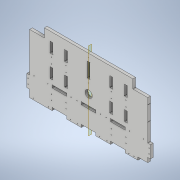
# Autodesk Inventor part: Side_one
Saved by Autodesk Inventor 2020 (Build 240168000, 168)
## iProperties
Created: 2019-12-17
Part Number: Side_one
Material: Generic
Document SubType Name: Modeling
Designer: fabfarm
Density: 1 g/cm^3
Appearance: Default
Author: fabfarm
Autodesk Inventor part; units mm, degrees
ref_plane "YZ Plane" through (0, 0, 0) normal (1, 0, 0) x (0, 1, 0)
ref_plane "XZ Plane" through (0, 0, 0) normal (0, 1, 0) x (-1, 0, 0)
ref_plane "XY Plane" through (0, 0, 0) normal (0, 0, 1) x (1, 0, 0)
sketch "Sketch1" plane through (0, 0, 0) normal (0, 0, 1) x (1, 0, 0)
  line L0 (0, 0) -> (-845, 0)
  line L1 (-845, 0) -> (-845, 464.3)
  line L2 (-845, 464.3) -> (0, 464.3)
  line L3 (0, 464.3) -> (0, 0)
  dimension "d0" = 464.3
  dimension "d1" = 845
  constraints: 8 end point, 2 parallel, 1 horizontal, 1 perpendicular
  measures "d0" distance of L2.end L0.start
  measures "d1" distance of L0.start L0.end
extrude "Extrusion1" add sketch "Sketch1" along normal blind 18.55
sketch "Sketch2" plane through (0, 0, 18.55) normal (0, 0, 1) x (1, 0, 0)
  line L0 (-845, 464.3) -> (-845, 0) projected
  line L1 (-845, 464.3) -> (-826.45, 464.3)
  line L2 (-826.45, 464.3) -> (-826.45, 359.9)
  line L3 (-826.45, 359.9) -> (-845, 359.9)
  line L4 (-845, 359.9) -> (-845, 464.3)
  line L5 (0, 464.3) -> (-845, 464.3) projected
  line L6 (-845, 259.9) -> (-826.45, 259.9)
  line L7 (-826.45, 259.9) -> (-826.45, 134.8)
  line L8 (-826.45, 134.8) -> (-845, 134.8)
  line L9 (-845, 134.8) -> (-845, 259.9)
  point P0 (-845, 359.9)
  point P1 (-845, 134.8)
  dimension "d54" = 18.55
  dimension "d55" = 104.4
  dimension "d86" = 100
  dimension "d87" = 125.1
  constraints: 16 end point, 4 parallel, 2 collinear, 2 horizontal, 2 perpendicular, 2 point on line
  measures "d54" distance of L1.start L1.end
  measures "d55" distance of L1.end L2.end
  measures "d86" distance between parallel lines of L6 L3
  measures "d87" distance of L6.end L7.end
extrude "Extrusion2" cut sketch "Sketch2" against normal blind 18.55
ref_plane "Work Plane1" through (-422.5, 259.9, 0) normal (-1, 0, 0) x (0, 0, 1)
mirror "Mirror1" about plane through (-422.5, 259.9, 0) normal (-1, 0, 0) of "Extrusion2"
sketch "Sketch3" plane through (0, 0, 18.55) normal (0, 0, 1) x (1, 0, 0)
  line L0 (0, 464.3) -> (-845, 464.3) projected
  line L1 (-845, 404.3) -> (-725, 404.3)
  line L2 (-725, 404.3) -> (-725, 464.3)
  line L3 (-725, 464.3) -> (-845, 464.3)
  line L4 (-845, 464.3) -> (-845, 404.3)
  point P0 (0, 0)
  point P1 (-18.55, 350)
  point P2 (0, 464.3)
  dimension "d19" = 120
  dimension "d22" = 60
  constraints: 8 end point, 2 perpendicular, 1 parallel, 2 other
  measures "d19" distance of L3.end L2.end
  measures "d22" distance of L3.end L1.start
extrude "Extrusion3" cut sketch "Sketch3" against normal blind 18.55
mirror "Mirror2" about plane through (-422.5, 259.9, 0) normal (-1, 0, 0) of "Extrusion3"
sketch "Sketch4" plane through (0, 0, 18.55) normal (0, 0, 1) x (1, 0, 0)
  line L0 (-672.5, 134.8) -> (-572.5, 134.8)
  line L1 (-572.5, 134.8) -> (-572.5, 153.35)
  line L2 (-572.5, 153.35) -> (-672.5, 153.35)
  line L3 (-672.5, 153.35) -> (-672.5, 134.8)
  line L4 (-472.5, 134.8) -> (-372.5, 134.8)
  line L5 (-372.5, 134.8) -> (-372.5, 153.35)
  line L6 (-372.5, 153.35) -> (-472.5, 153.35)
  line L7 (-472.5, 153.35) -> (-472.5, 134.8)
  line L8 (-272.5, 134.8) -> (-172.5, 134.8)
  line L9 (-172.5, 134.8) -> (-172.5, 153.35)
  line L10 (-172.5, 153.35) -> (-272.5, 153.35)
  line L11 (-272.5, 153.35) -> (-272.5, 134.8)
  line L12 (0, 0) -> (0, 359.9) projected
  line L13 (-845, 359.9) -> (-845, 0) projected
  line L14 (-826.45, 134.8) -> (-845, 134.8) projected
  line L15 (-845, 259.9) -> (-826.45, 259.9) projected
  line L16 (-120, 464.3) -> (-725, 464.3) projected
  line L17 (-422.5, 464.3) -> (-422.5, 153.35) construction
  dimension "d59" = 100
  dimension "d60" = 100
  dimension "d61" = 100
  dimension "d62" = 100
  dimension "d63" = 100
  dimension "d66" = 18.55
  constraints: 26 end point, 6 parallel, 5 collinear, 3 horizontal, 3 perpendicular, 2 midpoint, 1 vertical
  measures "d59" distance of L1.end L2.end
  measures "d60" distance of L5.end L6.end
  measures "d61" distance between parallel lines of L1 L7
  measures "d62" distance between parallel lines of L11 L5
  measures "d63" distance of L9.end L10.end
  measures "d66" distance of L2.end L0.start
extrude "Extrusion4" cut sketch "Sketch4" against normal blind 20
sketch "Sketch6" plane through (0, 0, 18.55) normal (0, 0, 1) x (1, 0, 0)
  line L0 (-372.5, 400.4) -> (-472.5, 400.4)
  line L1 (-472.5, 400.4) -> (-472.5, 425.4)
  line L2 (-472.5, 425.4) -> (-372.5, 425.4)
  line L3 (-372.5, 425.4) -> (-372.5, 400.4)
  line L4 (-372.5, 400.4) -> (-472.5, 425.4) construction
  line L5 (-472.5, 400.4) -> (-372.5, 425.4) construction
  line L6 (-422.5, -92.86) -> (-422.5, 557.16) projected
  line L7 (-120, 464.3) -> (-725, 464.3) projected
  point P0 (0, 0)
  point P1 (-422.5, 412.9)
  dimension "d38" = 25
  dimension "d39" = 100
  dimension "d40" = 38.9
  constraints: 12 end point, 2 midpoint, 2 parallel, 1 horizontal, 1 perpendicular, 1 point on line
  measures "d38" distance of L0.end L1.end
  measures "d39" distance of L1.end L2.end
  measures "d40" distance between parallel lines of L7 L2
extrude "Extrusion6" [suppressed]
fillet "Fillet1" [suppressed]
sketch "Sketch7" plane through (0, 0, 18.55) normal (0, 0, 1) x (1, 0, 0)
  line L0 (-686.45, 183.35) -> (-667.9, 183.35)
  line L1 (-667.9, 183.35) -> (-667.9, 253.85)
  line L2 (-667.9, 253.85) -> (-686.45, 253.85)
  line L3 (-686.45, 253.85) -> (-686.45, 183.35)
  line L4 (-586.5, 183.35) -> (-567.95, 183.35)
  line L5 (-567.95, 183.35) -> (-567.95, 253.85)
  line L6 (-567.95, 253.85) -> (-586.5, 253.85)
  line L7 (-586.5, 253.85) -> (-586.5, 183.35)
  line L8 (-725, 464.3) -> (-725, 404.3) projected
  line L9 (-672.5, 153.35) -> (-572.5, 153.35) projected
  line L10 (-826.45, 259.9) -> (-826.45, 134.8) projected
  point P0 (0, 0)
  dimension "d44" = 81.4
  dimension "d45" = 18.55
  dimension "d46" = 70.5
  dimension "d72" = 30
  dimension "d194" = 140
  constraints: 16 end point, 4 parallel, 2 horizontal, 2 perpendicular, 2 point on line, 1 collinear
  measures "d44" distance between parallel lines of L7 L1
  measures "d45" distance of L1.end L2.end
  measures "d46" distance of L2.end L0.start
  measures "d72" distance between parallel lines of L9 L0
  measures "d194" distance between parallel lines of L10 L3
extrude "Extrusion7" cut sketch "Sketch7" against normal blind 20
mirror "Mirror3" about plane through (-422.5, 259.9, 0) normal (-1, 0, 0) of "Extrusion7"
sketch "Esquisse8" plane through (0, 0, 0) normal (0, 0, -1) x (-1, 0, 0)
  line L0 (177.1, 334.35) -> (158.55, 334.35)
  line L1 (158.55, 334.35) -> (158.55, 404.85)
  line L2 (158.55, 404.85) -> (177.1, 404.85)
  line L3 (177.1, 404.85) -> (177.1, 334.35)
  line L4 (258.5, 404.85) -> (277.05, 404.85)
  line L5 (277.05, 404.85) -> (277.05, 334.35)
  line L6 (277.05, 334.35) -> (258.5, 334.35)
  line L7 (258.5, 334.35) -> (258.5, 404.85)
  line L8 (158.55, 183.35) -> (158.55, 253.85) projected
  line L9 (177.1, 253.85) -> (177.1, 183.35) projected
  line L10 (258.5, 183.35) -> (258.5, 253.85) projected
  line L11 (277.05, 253.85) -> (277.05, 183.35) projected
  line L12 (177.1, 253.85) -> (158.55, 253.85) projected
  point P0 (0, 0)
  dimension "d51" = 70.5
  dimension "d90" = 80.5
  constraints: 16 end point, 4 collinear, 4 parallel, 2 horizontal, 2 perpendicular, 2 point on line
  measures "d51" distance of L0.end L1.end
  measures "d90" distance between parallel lines of L0 L12
extrude "Extrusion8" cut sketch "Esquisse8" against normal blind 20
mirror "Symétrie4" about plane through (-422.5, 259.9, 0) normal (-1, 0, 0) of "Extrusion8"
sketch "Esquisse9" plane through (0, 0, 18.55) normal (0, 0, 1) x (1, 0, 0)
  circle A0 centre (-827.5708, 361.0208) radius 1.585
  circle A1 centre (-827.5708, 135.9208) radius 1.585
  circle A2 centre (-685.3292, 403.7292) radius 1.585
  circle A3 centre (-685.3292, 335.4708) radius 1.585
  circle A4 centre (-827.5708, 258.7792) radius 1.585
  circle A5 centre (-685.3292, 252.7292) radius 1.585
  circle A6 centre (-669.0208, 252.7292) radius 1.585
  circle A7 centre (-669.0208, 184.4708) radius 1.585
  circle A8 centre (-726.1208, 405.4208) radius 1.585
  circle A9 centre (-671.3792, 152.2292) radius 1.585
  circle A10 centre (-471.3792, 152.2292) radius 1.585
  line L0 (-120, 464.3) -> (-725, 464.3) projected
  line L1 (-422.5, 464.3) -> (-422.5, 151.8903) construction
  circle A11 centre (-671.3792, 135.9208) radius 1.585
  circle A12 centre (-471.3792, 135.9208) radius 1.585
  line L2 (-826.45, 359.9) -> (-827.5708, 361.0208) construction
  line L3 (-826.45, 404.3) -> (-826.45, 359.9) projected
  line L4 (-826.45, 259.9) -> (-827.5708, 258.7792) construction
  line L5 (-827.5708, 135.9208) -> (-826.45, 134.8) construction
  line L6 (-826.45, 259.9) -> (-826.45, 134.8) projected
  line L7 (-826.45, 404.3) -> (-725, 404.3) projected
  line L8 (-726.1208, 405.4208) -> (-725, 404.3) construction
  line L9 (-686.45, 404.85) -> (-685.3292, 403.7292) construction
  circle A13 centre (-666.7792, 335.4708) radius 1.585
  line L10 (-666.7792, 335.4708) -> (-667.9, 334.35) construction
  line L11 (-686.45, 334.35) -> (-685.3292, 335.4708) construction
  line L12 (-667.9, 334.35) -> (-686.45, 334.35) projected
  line L13 (-669.0208, 184.4708) -> (-667.9, 183.35) construction
  line L14 (-669.0208, 252.7292) -> (-667.9, 253.85) construction
  line L15 (-667.9, 253.85) -> (-667.9, 183.35) projected
  line L16 (-686.45, 183.35) -> (-685.3292, 184.4708) construction
  line L17 (-667.9, 183.35) -> (-686.45, 183.35) projected
  circle A14 centre (-685.3292, 184.4708) radius 1.585
  line L18 (-667.9, 334.35) -> (-667.9, 464.3) projected
  line L19 (-667.9, 411.8699) -> (-586.5, 369.6) construction
  line L20 (-586.5, 334.35) -> (-586.5, 404.85) construction
  line L21 (-627.2, 390.7349) -> (-626.3146, 152.6654) construction
  circle A15 centre (-569.169, 404.1612) radius 1.585
  circle A16 centre (-568.6613, 335.9046) radius 1.585
  circle A17 centre (-568.0459, 253.1654) radius 1.585
  circle A18 centre (-584.3539, 253.0441) radius 1.585
  circle A19 centre (-583.8463, 184.7875) radius 1.585
  line L22 (-568.0566, 405.2903) -> (-569.169, 404.1612) construction
  circle A20 centre (-587.2108, 335.7667) radius 1.585
  line L23 (-587.2108, 335.7667) -> (-586.5, 334.35) construction
  line L24 (-567.5323, 334.7922) -> (-568.6613, 335.9046) construction
  line L25 (-583.8463, 184.7875) -> (-584.9587, 183.6585) construction
  line L26 (-584.3539, 253.0441) -> (-585.483, 254.1565) construction
  line L27 (-566.4092, 183.7964) -> (-567.5382, 184.9088) construction
  circle A21 centre (-567.5382, 184.9088) radius 1.585
  line L28 (-586.5, 334.35) -> (-586.5, 404.85)
  line L29 (-586.6583, 412.172) -> (-667.7417, 369.2979) construction
  line L30 (-572.5, 134.8) -> (-672.5, 134.8) construction
  line L31 (-671.3792, 135.9208) -> (-672.5, 134.8) construction
  line L32 (-672.5, 153.35) -> (-572.5, 153.35) construction
  line L33 (-622.5, 153.35) -> (-622.5, 134.8) construction
  circle A22 centre (-573.6208, 152.2292) radius 1.585
  circle A23 centre (-573.6208, 135.9208) radius 1.585
  circle A24 centre (-17.4292, 361.0208) radius 1.585
  circle A25 centre (-17.4292, 135.9208) radius 1.585
  circle A26 centre (-176.0858, 403.632) radius 1.585
  line L34 (-159.6708, 403.7292) -> (-176.0858, 403.632) construction
  circle A27 centre (-159.6708, 403.7292) radius 1.585
  circle A28 centre (-159.6708, 335.4708) radius 1.585
  circle A29 centre (-17.4292, 258.7792) radius 1.585
  circle A30 centre (-159.6708, 252.7292) radius 1.585
  circle A31 centre (-175.9792, 252.7292) radius 1.585
  circle A32 centre (-175.9792, 184.4708) radius 1.585
  circle A33 centre (-118.8792, 405.4208) radius 1.585
  circle A34 centre (-173.6208, 152.2292) radius 1.585
  circle A35 centre (-373.6208, 152.2292) radius 1.585
  circle A36 centre (-173.6208, 135.9208) radius 1.585
  circle A37 centre (-373.6208, 135.9208) radius 1.585
  line L35 (-18.55, 359.9) -> (-17.4292, 361.0208) construction
  line L36 (-18.55, 404.3) -> (-18.55, 359.9)
  line L37 (-18.55, 259.9) -> (-17.4292, 258.7792) construction
  line L38 (-17.4292, 135.9208) -> (-18.55, 134.8) construction
  line L39 (-18.55, 259.9) -> (-18.55, 134.8)
  line L40 (-18.55, 404.3) -> (-120, 404.3)
  line L41 (-118.8792, 405.4208) -> (-120, 404.3) construction
  line L42 (-177.1, 404.85) -> (-158.55, 404.85)
  line L43 (-158.55, 404.85) -> (-159.6708, 403.7292) construction
  line L44 (-177.1, 404.85) -> (-176.0858, 403.632) construction
  circle A38 centre (-178.2208, 335.4708) radius 1.585
  line L45 (-178.2208, 335.4708) -> (-177.1, 334.35) construction
  line L46 (-158.55, 334.35) -> (-159.6708, 335.4708) construction
  line L47 (-177.1, 334.35) -> (-158.55, 334.35)
  line L48 (-175.9792, 184.4708) -> (-177.1, 183.35) construction
  line L49 (-175.9792, 252.7292) -> (-177.1, 253.85) construction
  line L50 (-177.1, 253.85) -> (-177.1, 183.35)
  line L51 (-158.55, 183.35) -> (-159.6708, 184.4708) construction
  line L52 (-177.1, 183.35) -> (-158.55, 183.35)
  circle A39 centre (-159.6708, 184.4708) radius 1.585
  line L53 (-177.1, 334.35) -> (-177.1, 404.85)
  line L54 (-177.1, 411.8699) -> (-258.5, 369.6) construction
  line L55 (-258.5, 334.35) -> (-258.5, 404.85) construction
  line L56 (-217.8, 390.7349) -> (-218.6854, 152.6654) construction
  circle A40 centre (-260.6461, 253.0441) radius 1.585
  circle A41 centre (-261.1537, 184.7875) radius 1.585
  circle A42 centre (-259.116, 404.064) radius 0.9986
  circle A43 centre (-276.9541, 253.1654) radius 1.585
  line L57 (-261.1537, 184.7875) -> (-260.0413, 183.6585) construction
  line L58 (-260.6461, 253.0441) -> (-259.517, 254.1565) construction
  line L59 (-278.5908, 183.7964) -> (-277.4618, 184.9088) construction
  circle A44 centre (-277.4618, 184.9088) radius 1.585
  line L60 (-275.831, 404.1612) -> (-259.116, 404.064) construction
  circle A45 centre (-276.3387, 335.9046) radius 1.585
  line L61 (-277.4677, 334.7922) -> (-276.3387, 335.9046) construction
  circle A46 centre (-257.7892, 335.7667) radius 1.585
  line L62 (-258.3417, 412.172) -> (-177.2583, 369.2979) construction
  line L63 (-258.5, 334.35) -> (-258.5, 404.85)
  line L64 (-257.7892, 335.7667) -> (-258.5, 334.35) construction
  circle A47 centre (-275.831, 404.1612) radius 1.585
  line L65 (-276.9434, 405.2903) -> (-275.831, 404.1612) construction
  line L66 (-258.5, 404.85) -> (-259.116, 404.064) construction
  line L67 (-272.5, 134.8) -> (-172.5, 134.8) construction
  line L68 (-173.6208, 135.9208) -> (-172.5, 134.8) construction
  line L69 (-172.5, 153.35) -> (-272.5, 153.35) construction
  line L70 (-222.5, 153.35) -> (-222.5, 134.8) construction
  circle A48 centre (-271.3792, 152.2292) radius 1.585
  circle A49 centre (-271.3792, 135.9208) radius 1.585
  line L71 (-686.45, 404.85) -> (-667.9, 404.85) projected
  circle A50 centre (-669.0208, 403.7292) radius 1.585
  line L72 (-667.9, 404.85) -> (-669.0208, 403.7292) construction
  circle A51 centre (-585.477, 404.0399) radius 1.585
  point P0 (-567.95, 183.35)
  point P1 (-372.5, 153.35)
  point P2 (-567.95, 404.85)
  point P3 (-258.5, 334.35)
  point P4 (-472.5, 134.8)
  point P5 (-272.5, 153.35)
  point P6 (-277.05, 183.35)
  point P7 (-277.05, 404.85)
  point P8 (-172.5, 153.35)
  point P9 (-372.5, 134.8)
  dimension "d69" = 3.17
  dimension "d115" = 45
  dimension "d117" = 45
  dimension "d118" = 45
  dimension "d119" = 45
  dimension "d123" = 45
  dimension "d129" = 45
  dimension "d130" = 45
  dimension "d131" = 45
  dimension "d132" = 45
  dimension "d143" = 45
  dimension "d144" = 45
  constraints: 116 end point, 86 symmetric about line, 20 vertical, 14 coincident, 11 centre point, 5 horizontal alignment, 4 midpoint, 3 vertical alignment, 154 other
  measures "d115" angle of L3 L2
  measures "d117" angle of L6 L5
  measures "d118" angle of L6 L4
  measures "d119" angle of L7 L8
  measures "d123" angle of L12 L11
  measures "d129" angle of L15 L14
  measures "d130" angle of L15 L13
  measures "d131" angle of L17 L16
  measures "d132" angle of L30 L31
  measures "d143" angle of L9 L71
  measures "d144" angle to the sketch x axis of L72
extrude "Extrusion9" cut sketch "Esquisse9" against normal blind 20
sketch "Esquisse11" plane through (0, 0, 18.55) normal (0, 0, 1) x (1, 0, 0)
  circle A0 centre (-835.725, 329.9) radius 2.25
  circle A1 centre (-835.725, 289.9) radius 2.25
  circle A2 centre (-677.175, 314.35) radius 2.25
  circle A3 centre (-677.175, 273.85) radius 2.25
  circle A4 centre (-577.225, 314.35) radius 2.25
  circle A5 centre (-577.225, 273.85) radius 2.25
  line L0 (-667.9, 334.35) -> (-686.45, 334.35) projected
  line L1 (-677.175, 334.35) -> (-677.175, 253.85) construction
  line L2 (-686.45, 253.85) -> (-667.9, 253.85) projected
  line L3 (-567.95, 334.35) -> (-586.5, 334.35) projected
  line L4 (-577.225, 334.35) -> (-577.225, 253.85) construction
  line L5 (-586.5, 253.85) -> (-567.95, 253.85) projected
  line L6 (-826.45, 359.9) -> (-845, 359.9) projected
  line L7 (-120, 464.3) -> (-725, 464.3) projected
  line L8 (-422.5, 464.3) -> (-422.5, 153.35) construction
  line L9 (-472.5, 153.35) -> (-372.5, 153.35) projected
  circle A6 centre (-9.275, 329.9) radius 2.25
  circle A7 centre (-9.275, 289.9) radius 2.25
  circle A8 centre (-167.825, 314.35) radius 2.25
  circle A9 centre (-167.825, 273.85) radius 2.25
  circle A10 centre (-267.775, 314.35) radius 2.25
  circle A11 centre (-267.775, 273.85) radius 2.25
  line L10 (-167.825, 334.35) -> (-167.825, 253.85) construction
  line L11 (-160.7915, 253.85) -> (-174.8585, 253.85)
  line L12 (-371.265, 334.65) -> (-355.585, 334.65)
  line L13 (-267.775, 334.35) -> (-267.775, 253.85) construction
  line L14 (-355.585, 253.65) -> (-371.265, 253.65)
  line L15 (-16.3085, 359.9) -> (0, 359.9)
  line L16 (-845, 259.9) -> (-826.45, 259.9) projected
  line L17 (-835.725, 359.9) -> (-835.725, 259.9) construction
  point P0 (-573.5723, 199.8)
  point P1 (-684.2085, 334.35)
  point P2 (-684.2085, 253.85)
  point P3 (-670.1415, 253.85)
  point P4 (-473.735, 334.65)
  point P5 (-489.415, 334.65)
  point P6 (-489.415, 253.65)
  point P7 (-473.735, 253.65)
  point P8 (-828.6915, 359.9)
  point P9 (-470.2585, 153.35)
  point P10 (-277.485, 153.35)
  point P11 (-355.585, 253.65)
  point P12 (-371.265, 253.65)
  point P13 (-828.6915, 259.9)
  point P14 (-686.45, 334.35)
  point P15 (-567.95, 253.85)
  dimension "d76" = 4.5
  dimension "d79" = 30
  dimension "d80" = 20
  dimension "d81" = 20
  dimension "d82" = 20
  dimension "d83" = 20
  dimension "d91" = 30
  constraints: 18 symmetric about line, 16 end point, 12 centre point, 10 point on line, 5 equal radius, 5 midpoint, 18 other
  measures "d76" diameter of A0
  measures "d79" distance from line of L6 A0.centre
  measures "d80" distance from line of L2 A3.centre
  measures "d91" distance from line of A1.centre L16
extrude "Extrusion10" cut sketch "Esquisse11" against normal blind 20
sketch "Esquisse12" plane through (0, 0, 18.55) normal (0, 0, 1) x (1, 0, 0)
  line L0 (-845, 0) -> (0, 0) projected
  line L1 (-672.5, 0) -> (-572.5, 0)
  line L2 (-572.5, 0) -> (-572.5, 18.55)
  line L3 (-572.5, 18.55) -> (-672.5, 18.55)
  line L4 (-672.5, 18.55) -> (-672.5, 0)
  line L5 (-472.5, 0) -> (-372.5, 0)
  line L6 (-372.5, 0) -> (-372.5, 18.55)
  line L7 (-372.5, 18.55) -> (-472.5, 18.55)
  line L8 (-472.5, 18.55) -> (-472.5, 0)
  line L9 (-272.5, 0) -> (-172.5, 0)
  line L10 (-172.5, 0) -> (-172.5, 18.55)
  line L11 (-172.5, 18.55) -> (-272.5, 18.55)
  line L12 (-272.5, 18.55) -> (-272.5, 0)
  line L13 (-572.5, 153.35) -> (-572.5, 134.8) projected
  line L14 (-672.5, 134.8) -> (-672.5, 153.35) projected
  line L15 (-472.5, 134.8) -> (-472.5, 153.35) projected
  line L16 (-372.5, 153.35) -> (-372.5, 134.8) projected
  line L17 (-272.5, 134.8) -> (-272.5, 153.35) projected
  line L18 (-172.5, 153.35) -> (-172.5, 134.8) projected
  point P0 (-475.9, 151.865)
  point P1 (-475.9, 136.385)
  point P2 (-672.5, 137.0415)
  point P3 (-672.5, 151.1085)
  point P4 (-472.5, 137.0415)
  point P5 (-472.5, 151.1085)
  point P6 (-275.9, 151.865)
  point P7 (-275.9, 136.385)
  point P8 (-176.1, 136.385)
  point P9 (-176.1, 151.865)
  point P10 (-75.9, 151.865)
  point P11 (-75.9, 136.385)
  point P12 (-172.5, 0)
  point P13 (-572.5, 0)
  point P14 (-372.5, 0)
  point P15 (-372.5, 134.8)
  dimension "d92" = 18.55
  constraints: 24 end point, 6 parallel, 4 point on line, 4 vertical, 3 collinear, 3 horizontal, 3 perpendicular, 4 other
  measures "d92" distance of L3.end L1.start
extrude "Extrusion11" cut sketch "Esquisse12" against normal blind 20
sketch "Esquisse13" plane through (0, 0, 18.55) normal (0, 0, 1) x (1, 0, 0)
  circle A0 centre (-671.3686, 17.4186) radius 1.6
  line L0 (-672.5, 0) -> (-672.5, 18.55) construction
  line L1 (-672.5, 18.55) -> (-671.3686, 17.4186) construction
  line L2 (-672.5, 18.55) -> (-572.5, 18.55) projected
  circle A1 centre (-573.6314, 17.4186) radius 1.6
  circle A2 centre (-471.3686, 17.4186) radius 1.6
  line L3 (-422.5, 18.55) -> (-422.5, 134.8) construction
  line L4 (-372.5, 134.8) -> (-472.5, 134.8) projected
  line L5 (-472.5, 18.55) -> (-372.5, 18.55) projected
  circle A3 centre (-173.6314, 17.4186) radius 1.6
  line L6 (-172.5, 0) -> (-172.5, 18.55) construction
  line L7 (-172.5, 18.55) -> (-173.6314, 17.4186) construction
  line L8 (-172.5, 18.55) -> (-272.5, 18.55) construction
  circle A4 centre (-271.3686, 17.4186) radius 1.6
  circle A5 centre (-373.6314, 17.4186) radius 1.6
  point P0 (0, 0)
  point P1 (-272.5, 18.55)
  point P2 (-172.5, 18.55)
  point P3 (-374.7415, 134.8)
  point P4 (-470.2585, 134.8)
  point P5 (-270.2373, 18.55)
  point P6 (-574.7627, 18.55)
  dimension "d95" = 3.2
  dimension "d133" = 45
  constraints: 10 end point, 6 symmetric about line, 4 vertical, 2 horizontal alignment, 2 midpoint, 18 other
  measures "d133" angle of L2 L1
extrude "Extrusion12" cut sketch "Esquisse13" against normal blind 20
sketch "Esquisse14" plane through (0, 0, 18.55) normal (0, 0, 1) x (1, 0, 0)
  circle A0 centre (-677.175, 94.8) radius 2.25
  circle A1 centre (-677.175, 58.55) radius 2.25
  circle A2 centre (-577.225, 94.8) radius 2.25
  circle A3 centre (-577.225, 58.55) radius 2.25
  line L0 (-667.9, 183.35) -> (-686.45, 183.35) projected
  line L1 (-677.175, 183.35) -> (-677.175, 0) construction
  line L2 (-845, 0) -> (-672.5, 0) projected
  line L3 (-567.95, 183.35) -> (-586.5, 183.35) projected
  line L4 (-577.225, 183.35) -> (-577.225, -0.1) construction
  line L5 (-670.2373, 18.55) -> (-572.5, 18.55) projected
  line L6 (-572.5, 134.8) -> (-672.5, 134.8) projected
  line L7 (-472.5, 18.55) -> (-372.5, 18.55) projected
  line L8 (-422.5, 18.55) -> (-422.5, 134.8) construction
  line L9 (-372.5, 134.8) -> (-472.5, 134.8) projected
  circle A4 centre (-167.825, 94.8) radius 2.25
  circle A5 centre (-167.825, 58.55) radius 2.25
  circle A6 centre (-267.775, 94.8) radius 2.25
  circle A7 centre (-267.775, 58.55) radius 2.25
  point P0 (0, 0)
  point P1 (-477.5, 18.55)
  point P2 (-477.485, 134.8)
  point P3 (-670.2585, 134.8)
  point P4 (-374.5, 18.55)
  point P5 (-277.5, 18.55)
  point P6 (-277.485, 134.8)
  point P7 (-470.2585, 134.8)
  dimension "d98" = 4.5
  dimension "d99" = 40
  dimension "d100" = 40
  dimension "d101" = 40
  dimension "d103" = 40
  constraints: 8 centre point, 6 end point, 5 point on line, 4 midpoint, 4 symmetric about line, 3 equal radius, 2 vertical, 4 other
  measures "d98" diameter of A0
  measures "d99" distance from line of L5 A3.centre
  measures "d100" distance from line of L6 A2.centre
  measures "d101" distance from line of L6 A0.centre
  measures "d103" distance from line of L5 A1.centre
extrude "Extrusion13" cut sketch "Esquisse14" against normal blind 20
sketch "Esquisse16" plane through (0, 0, 18.55) normal (0, 0, 1) x (1, 0, 0)
  line L0 (0, 0) -> (0, 134.8) projected
  line L1 (-172.5, 0) -> (0, 0) projected
  line L2 (0, 50) -> (-18.55, 50)
  line L3 (-18.55, 50) -> (-18.55, 0)
  line L4 (-18.55, 0) -> (0, 0)
  line L5 (0, 0) -> (0, 50)
  line L6 (-18.55, 134.8) -> (-18.55, 259.9) projected
  line L7 (0, 134.8) -> (-18.55, 134.8) projected
  line L8 (-845, 0) -> (-672.5, 0) projected
  line L9 (-845, 50) -> (-826.45, 50)
  line L10 (-826.45, 50) -> (-826.45, 0)
  line L11 (-826.45, 0) -> (-845, 0)
  line L12 (-845, 0) -> (-845, 50)
  line L13 (-826.45, 259.9) -> (-826.45, 134.8) projected
  line L14 (-845, 134.8) -> (-845, 0) projected
  point P0 (-18.55, 136.385)
  point P1 (-18.55, 258.315)
  point P2 (-16.965, 134.8)
  dimension "d110" = 50
  dimension "d111" = 84.8
  constraints: 16 end point, 4 collinear, 4 parallel, 3 point on line, 2 horizontal, 2 perpendicular
  measures "d110" distance of L2.end L3.end
  measures "d111" distance between parallel lines of L7 L2
extrude "Extrusion15" cut sketch "Esquisse16" against normal blind 60
sketch "Esquisse18" plane through (0, 0, 18.55) normal (0, 0, 1) x (1, 0, 0)
  line L0 (-826.45, 50) -> (-826.45, 0) projected
  circle A0 centre (-827.5814, 48.8686) radius 1.6
  circle A1 centre (-17.4186, 48.8686) radius 1.6
  line L1 (-18.55, 50) -> (0, 50) construction
  line L2 (-18.55, 50) -> (-17.4186, 48.8686) construction
  line L3 (-18.55, 0) -> (-18.55, 50) construction
  point P0 (0, 0)
  dimension "d136" = 3.2
  dimension "d135" = 45
  constraints: 2 end point, 1 horizontal alignment, 6 other
  measures "d135" angle of L3 L2
extrude "Extrusion16" cut sketch "Esquisse18" against normal blind 20
sketch "Esquisse17" plane through (0, 0, 18.55) normal (0, 0, 1) x (1, 0, 0)
  circle A0 centre (-8.9415, 109.8) radius 2.25
  circle A1 centre (-8.9415, 75) radius 2.25
  circle A2 centre (-836.5228, 109.8) radius 2.25
  circle A3 centre (-836.5228, 75) radius 2.25
  line L0 (-845, 134.8) -> (-826.45, 134.8) projected
  line L1 (-835.725, 134.8) -> (-836.8564, 50) construction
  line L2 (-828.7127, 50) -> (-845, 50) projected
  line L3 (-18.55, 134.8) -> (0, 134.8) construction
  line L4 (-9.275, 134.8) -> (-8.1436, 50) construction
  line L5 (-16.2873, 50) -> (0, 50) construction
  point P0 (0, 0)
  point P1 (-828.6915, 134.8)
  point P2 (-16.3085, 134.8)
  dimension "d134" = 4.5
  dimension "d139" = 25
  dimension "d140" = 25
  constraints: 4 centre point, 4 end point, 4 midpoint, 3 equal radius, 2 horizontal alignment, 2 point on line, 2 vertical alignment
  measures "d134" diameter of A2
  measures "d139" distance from line of L0 A2.centre
  measures "d140" distance from line of A3.centre L2
extrude "Extrusion17" cut sketch "Esquisse17" against normal blind 20
sketch "Esquisse19" plane through (0, 0, 18.55) normal (0, 0, 1) x (1, 0, 0)
  line L0 (-567.95, 403.1482) -> (-567.95, 337.3211) projected
  line L1 (-413.225, 314.3) -> (-431.775, 314.3)
  line L2 (-431.775, 314.3) -> (-431.775, 414.3)
  line L3 (-431.775, 414.3) -> (-413.225, 414.3)
  line L4 (-413.225, 414.3) -> (-413.225, 314.3)
  line L5 (-120, 464.3) -> (-725, 464.3) projected
  line L6 (-422.5, 464.3) -> (-422.5, 414.3) construction
  point P0 (0, 0)
  point P1 (-558.95, 404.5204)
  dimension "d169" = 100
  dimension "d170" = 18.55
  dimension "d171" = 50
  constraints: 10 end point, 2 midpoint, 2 parallel, 1 horizontal, 1 perpendicular, 1 vertical, 1 other
  measures "d169" distance of L3.end L1.start
  measures "d170" distance of L1.start L1.end
  measures "d171" distance between parallel lines of L5 L3
extrude "Extrusion18" cut sketch "Esquisse19" against normal blind 18.55
sketch "Esquisse20" plane through (0, 0, 18.55) normal (0, 0, 1) x (1, 0, 0)
  line L0 (0, 259.9) -> (-18.55, 259.9)
  line L1 (-18.55, 259.9) -> (-18.55, 359.9)
  line L2 (-18.55, 359.9) -> (0, 359.9)
  line L3 (0, 359.9) -> (0, 259.9)
  line L4 (-826.45, 137.0415) -> (-826.45, 257.6585) projected
  line L5 (-826.45, 259.9) -> (-845, 259.9)
  line L6 (-845, 259.9) -> (-845, 359.9)
  line L7 (-845, 359.9) -> (-826.45, 359.9)
  line L8 (-826.45, 359.9) -> (-826.45, 259.9)
  line L9 (0, 359.9) -> (-18.55, 359.9) projected
  line L10 (-845, 359.9) -> (-845, 259.9) projected
  line L11 (-18.55, 359.9) -> (-18.55, 404.3) projected
  point P0 (0, 0)
  point P1 (-16.3085, 359.9)
  point P2 (-18.55, 362.1415)
  constraints: 16 end point, 5 collinear, 4 parallel, 2 horizontal, 2 perpendicular, 1 point on line
extrude "Extrusion19" cut sketch "Esquisse20" against normal blind 18.55
sketch "Esquisse21" plane through (0, 0, 18.55) normal (0, 0, 1) x (1, 0, 0)
  circle A0 centre (-422.5, 223.35) radius 25
  line L0 (-470.2585, 153.35) -> (-372.5, 153.35) projected
  line L1 (-422.5, 223.35) -> (-422.5, 464.3) construction
  line L2 (-120, 464.3) -> (-725, 464.3) projected
  point P0 (0, 0)
  dimension "d157" = 50
  dimension "d191" = 70
  constraints: 2 end point, 1 centre point, 1 midpoint, 1 vertical
  measures "d157" diameter of A0
  measures "d191" distance from line of L0 L1.start
extrude "Extrusion20" cut sketch "Esquisse21" against normal blind 18.55
sketch "Esquisse22" plane through (0, 0, 18.55) normal (0, 0, 1) x (1, 0, 0)
  circle A0 centre (-347.5, 9) radius 2.25
  circle A1 centre (-297.5, 9) radius 2.25
  circle A2 centre (-547.5, 9) radius 2.25
  circle A3 centre (-497.5, 9) radius 2.25
  line L0 (-572.5, 16.2873) -> (-572.5, 0) projected
  line L1 (-472.5, 0) -> (-472.5, 16.2873) projected
  line L2 (-372.5, 16.2873) -> (-372.5, 0) projected
  line L3 (-272.5, 0) -> (-272.5, 16.2873) projected
  line L4 (-372.5, 0) -> (-272.5, 0) projected
  circle A4 centre (-697.5, 9) radius 2.25
  circle A5 centre (-801.45, 9) radius 2.25
  line L5 (-672.5, 0) -> (-672.5, 16.2873) projected
  line L6 (-826.45, 47.7373) -> (-826.45, 0) projected
  circle A6 centre (-147.5, 9) radius 2.25
  circle A7 centre (-112.5, 9) radius 2.25
  line L7 (-172.5, 16.2873) -> (-172.5, 0) projected
  line L8 (-18.55, 0) -> (-18.55, 47.7373) projected
  point P0 (0, 0)
  dimension "d161" = 25
  dimension "d162" = 25
  dimension "d163" = 25
  dimension "d164" = 25
  dimension "d165" = 4.5
  dimension "d166" = 9
  dimension "d195" = 25
  dimension "d196" = 25
  dimension "d197" = 25
  dimension "d205" = 35
  constraints: 8 centre point, 7 equal radius, 7 horizontal alignment
  measures "d161" distance from line of L0 A2.centre
  measures "d162" distance from line of L1 A3.centre
  measures "d163" distance from line of L2 A0.centre
  measures "d164" distance from line of L3 A1.centre
  measures "d165" diameter of A0
  measures "d166" distance from line of L4 A0.centre
  measures "d195" distance from line of L5 A4.centre
  measures "d196" distance from line of L6 A5.centre
  measures "d197" distance from line of A6.centre L7
  measures "d205" distance of A7.centre A6.centre
extrude "Extrusion21" cut sketch "Esquisse22" against normal blind 20
sketch "Esquisse24" plane through (0, 0, 18.55) normal (0, 0, 1) x (1, 0, 0)
  circle A0 centre (-430.6436, 413.1686) radius 1.6
  circle A1 centre (-414.3564, 413.1686) radius 1.6
  circle A2 centre (-430.6436, 315.4314) radius 1.6
  line L0 (-413.225, 414.3) -> (-413.225, 314.3) projected
  circle A3 centre (-414.3564, 315.4314) radius 1.6
  line L1 (-431.775, 314.3) -> (-431.775, 414.3) projected
  line L2 (-431.775, 414.3) -> (-430.6436, 413.1686) construction
  circle A4 centre (-422.5, 289.3) radius 2.25
  line L3 (-431.775, 314.3) -> (-413.225, 314.3) projected
  line L4 (-422.5, 314.3) -> (-422.5, 289.3) construction
  circle A5 centre (-422.45, 439.3) radius 2.25
  line L5 (-431.775, 414.3) -> (-413.225, 414.3) projected
  point P0 (0, 0)
  dimension "d173" = 3.2
  dimension "d174" = 45
  dimension "d175" = 4.5
  dimension "d176" = 25
  dimension "d177" = 25
  dimension "d178" = 4.5
  dimension "d179" = 9.325
  constraints: 4 end point, 3 centre point, 2 horizontal alignment, 2 vertical alignment, 1 midpoint, 1 vertical, 12 other
  measures "d174" angle of L1 L2
  measures "d175" diameter of A4
  measures "d176" distance of L4.start L4.end
  measures "d177" distance from line of L5 A5.centre
  measures "d178" diameter of A5
  measures "d179" distance from line of L1 A5.centre
extrude "Extrusion22" cut sketch "Esquisse24" against normal blind 18.55 contours A0 L1 L5 | L5 A0 | A0 L1 | L5 L0 A1 | A1 L5 | L1 A2 | A2 L3 L1 | A1 L0 | L3 A2 | A3 L0 | L0 L3 A3 | A3 L3 | A4 | A5
sketch "Esquisse25" plane through (0, 0, 18.55) normal (0, 0, 1) x (1, 0, 0)
  line L0 (-572.5, 151.1085) -> (-572.5, 137.0415) projected
  line L1 (-572.5, 144.075) -> (-472.5, 144.075) construction
  line L2 (-472.5, 137.0415) -> (-472.5, 151.1085) projected
  circle A0 centre (-542.5, 144.075) radius 2.25
  circle A1 centre (-502.5, 144.075) radius 2.25
  circle A2 centre (-342.5, 144.075) radius 2.25
  circle A3 centre (-302.5, 144.075) radius 2.25
  circle A4 centre (-142.5, 144.075) radius 2.25
  circle A5 centre (-702.5, 144.075) radius 2.25
  line L3 (-672.5, 137.0415) -> (-672.5, 151.1085) projected
  line L4 (-172.5, 153.35) -> (-172.5, 134.8) projected
  line L5 (-272.5, 134.8) -> (-272.5, 153.35) projected
  line L6 (-372.5, 153.35) -> (-372.5, 134.8) projected
  circle A6 centre (-796.45, 144.075) radius 2.25
  circle A7 centre (-48.55, 144.075) radius 2.25
  line L7 (-826.45, 257.6585) -> (-826.45, 137.0415) projected
  line L8 (-18.55, 137.0415) -> (-18.55, 257.6585) projected
  point P0 (0, 0)
  point P1 (-172.5, 151.1085)
  point P2 (-172.5, 137.0415)
  point P3 (-272.5, 137.0415)
  point P4 (-272.5, 151.1085)
  point P5 (-372.5, 151.1085)
  point P6 (-372.5, 137.0415)
  dimension "d182" = 30
  dimension "d183" = 30
  dimension "d184" = 30
  dimension "d185" = 30
  dimension "d186" = 30
  dimension "d187" = 30
  dimension "d188" = 4.5
  dimension "d192" = 30
  dimension "d193" = 30
  constraints: 8 centre point, 7 equal radius, 7 horizontal alignment, 2 end point, 2 midpoint, 2 point on line, 1 horizontal
  measures "d182" distance from line of L3 A5.centre
  measures "d183" distance from line of L4 A4.centre
  measures "d184" distance from line of L5 A3.centre
  measures "d185" distance from line of L6 A2.centre
  measures "d186" horizontal distance of L2.start A1.centre
  measures "d187" distance from line of L0 A0.centre
  measures "d188" diameter of A1
  measures "d192" distance from line of A6.centre L7
  measures "d193" distance from line of L8 A7.centre
extrude "Extrusion23" cut sketch "Esquisse25" against normal blind 30
sketch "Esquisse26" plane through (0, 0, 18.55) normal (0, 0, 1) x (1, 0, 0)
  line L0 (-18.55, 47.7373) -> (-18.55, 0) projected
  line L1 (-18.55, 0) -> (-85, 0)
  line L2 (-85, 0) -> (-85, 16.2873)
  line L3 (-82.7373, 18.55) -> (-18.55, 18.55)
  line L4 (-18.55, 18.55) -> (-18.55, 0)
  line L5 (-85, 18.55) -> (-83.8686, 17.4186) construction
  arc A0 (-82.7373, 18.55) -> (-85, 16.2873) centre (-83.8686, 17.4186) ccw
  line L6 (-270.2373, 18.55) -> (-174.7627, 18.55) projected
  line L7 (0, 50) -> (0, 134.8) projected
  point P0 (0, 0)
  dimension "d199" = 45
  dimension "d200" = 3.2
  dimension "d204" = 85
  constraints: 10 end point, 3 point on circle, 2 parallel, 2 point on line, 1 centre point, 1 coincident, 1 collinear, 1 horizontal, 1 perpendicular
  measures "d199" angle of L3 L5
  measures "d200" diameter of A0
  measures "d204" distance between parallel lines of L7 L2
extrude "Extrusion24" cut sketch "Esquisse26" against normal blind 20
body "Solid1"
